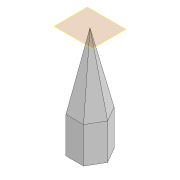
# Autodesk Inventor part: Punta caibración
Saved by Autodesk Inventor 2022 (Build 260153000, 153)
## iProperties
Created: 2022-11-09
Part Number: Punta caibración
Material: Generic
Document SubType Name: Modeling
Designer: ADMIN
Density: 1 g/cm^3
Appearance: Default
Author: ADMIN
## iProperties of the stored document Punta caibración_3DPrint.ipt
Created: 2022-11-09
Part Number: Punta caibración_3DPrint
Material: Generic
Document SubType Name: Modeling
Designer: ADMIN
Density: 1 g/cm^3
Appearance: Default
Author: ADMIN
Autodesk Inventor part; units mm, degrees
ref_plane "YZ Plane" through (0, 0, 0) normal (1, 0, 0) x (0, 1, 0)
ref_plane "XZ Plane" through (0, 0, 0) normal (0, 1, 0) x (-1, 0, 0)
ref_plane "XY Plane" through (0, 0, 0) normal (0, 0, 1) x (1, 0, 0)
sketch "Sketch1" plane through (0, 0, 0) normal (0, 1, 0) x (-1, 0, 0)
  line L0 (-4.9075, -8.5) -> (-9.815, 0)
  line L1 (-9.815, 0) -> (-4.9075, 8.5)
  line L2 (-4.9075, 8.5) -> (4.9075, 8.5)
  line L3 (4.9075, 8.5) -> (9.815, 0)
  line L4 (9.815, 0) -> (4.9075, -8.5)
  line L5 (4.9075, -8.5) -> (-4.9075, -8.5)
  point P0 (0, 0)
  point P1 (0, 0)
  dimension "d0" = 17
  constraints: 12 end point, 1 coincident, 13 other
  measures "d0" distance between parallel lines of L5 L2
extrude "Extrusion1" add sketch "Sketch1" along normal blind 20
ref_plane "Work Plane1" through (0, 60, 0) normal (0, 1, 0) x (1, 0, 0)
sketch "Sketch2" plane through (0, 60, 0) normal (0, 1, 0) x (1, 0, 0)
  point P0 (0, 0)
  point P1 (0, 0)
  constraints: 1 coincident
loft "Loft1" add section 1 edges at (-7.3612, 20, -4.25) (-7.3612, 20, 4.25) (0, 20, 8.5) (7.3612, 20, 4.25) (7.3612, 20, -4.25) (0, 20, -8.5) section 2 point at (0, 60, 0)
body "Solid1"
